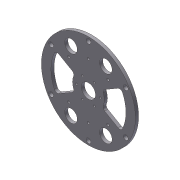
# Autodesk Inventor part: FlyWheel_Base_Jan21
Saved by Autodesk Inventor 2012 (Build 160160000, 160)
## iProperties
Created: 2012-01-22
Part Number: FlyWheel_Base_Jan21
Material: Aluminum-6061
Document SubType Name: Modeling
Designer: JesseK
Density: 2.71 g/cm^3
Mass: 341.466 g
Surface Area: 506.466 cm^2
Volume: 126.002 cm^3
Author: JesseK
Autodesk Inventor part; units mm, degrees
ref_plane "YZ Plane" through (0, 0, 0) normal (1, 0, 0) x (0, 1, 0)
ref_plane "XZ Plane" through (0, 0, 0) normal (0, 1, 0) x (-1, 0, 0)
ref_plane "XY Plane" through (0, 0, 0) normal (0, 0, 1) x (1, 0, 0)
sketch "Sketch1" plane through (0, 0, 0) normal (0, 0, 1) x (1, 0, 0)
  circle A0 centre (0, 0) radius 94.2975
  circle A1 centre (0, 0) radius 14.2875
  dimension "d0" = 188.595
  dimension "d1" = 28.575
  constraints: 2 centre point, 2 coincident
  measures "d0" diameter of A0
  measures "d1" diameter of A1
extrude "Extrusion1" add sketch "Sketch1" along normal blind 6.35
sketch "Sketch2" plane through (0, 0, 6.35) normal (0, 0, 1) x (1, 0, 0)
  circle A0 centre (0, 0) radius 94.2975 projected
  circle A1 centre (0, 0) radius 23.8125 construction
  line L0 (0, 0) -> (-11.9063, 20.6222) construction
  line L1 (0, 0) -> (0, 23.8125) construction
  circle A2 centre (-11.9063, 20.6222) radius 2.0193
  dimension "d4" = 47.625
  dimension "d5" = 30
  dimension "d6" = 4.0386
  constraints: 4 end point, 2 centre point, 2 coincident, 2 point on circle, 1 vertical
  measures "d4" diameter of A1
  measures "d5" angle of L1 L0
  measures "d6" diameter of A2
extrude "Extrusion2" cut sketch "Sketch2" against normal through all contours A2
pattern_circular "Circular Pattern1" count 6 over 360 about axis through (0, 0, -10) along (0, 0, 1) of "Extrusion2"
sketch "Sketch6" plane through (0, 0, 0) normal (0, 0, -1) x (-1, 0, 0)
  circle A0 centre (0, 0) radius 94.2975 projected
  circle A1 centre (0, 0) radius 55.5625 construction
  line L0 (0, 0) -> (0, -55.5625) construction
  circle A2 centre (0, -55.5625) radius 2.4384
  circle A3 centre (0, 0) radius 14.2875 projected
  line L1 (0, 0) -> (-39.2886, -39.2886) construction
  line L2 (0, 0) -> (39.2886, -39.2886) construction
  circle A4 centre (-39.2886, -39.2886) radius 2.4384
  circle A5 centre (39.2886, -39.2886) radius 2.4384
  dimension "d32" = 111.125
  dimension "d37" = 45
  dimension "d38" = 4.8768
  constraints: 6 end point, 4 centre point, 4 coincident, 3 point on circle, 2 equal radius, 1 perpendicular, 1 vertical
  measures "d32" diameter of A1
  measures "d37" angle of L0 L1
  measures "d38" diameter of A2
extrude "Extrusion5" cut sketch "Sketch6" against normal up to next contours A2 | A4 | A5
pattern_circular "Circular Pattern4" count 2 over 360 about axis through (0, 0, -10) along (0, 0, 1) of "Extrusion5"
sketch "Sketch7" plane through (0, 0, 0) normal (0, 0, -1) x (-1, 0, 0)
  circle A0 centre (0, 0) radius 94.2975 projected
  circle A1 centre (0, 0) radius 86.5188 construction
  circle A2 centre (0, -86.5188) radius 4.7625
  line L0 (0, -86.5188) -> (0, 0) construction
  dimension "d42" = 173.0375
  dimension "d43" = 9.525
  constraints: 2 end point, 1 centre point, 1 coincident, 1 vertical, 1 vertical alignment, 2 other
  measures "d43" diameter of A2
extrude "Extrusion6" cut sketch "Sketch7" against normal through all contours A2
pattern_circular "Circular Pattern5" count 6 over 360 about axis through (0, 0, -10) along (0, 0, 1) of "Extrusion6"
sketch "Sketch8" plane through (0, 0, 0) normal (0, 0, -1) x (-1, 0, 0)
  circle A0 centre (0, 0) radius 94.2975 projected
  arc A1 (-29.7576, 11.0702) -> (-29.7576, -11.0702) centre (0, 0) ccw
  arc A2 (-68.3565, 31.4575) -> (-68.3565, -31.4575) centre (0, 0) ccw
  line L0 (-59.413, 34.3021) -> (-32.5341, 18.7836)
  line L1 (-59.413, -34.3021) -> (-32.5341, -18.7836)
  line L2 (-27.4963, -15.875) -> (0, 0) construction
  line L3 (0, 0) -> (-27.4963, 15.875) construction
  line L4 (0, 0) -> (-75.2475, 0) construction
  line L5 (-65.1662, 37.6237) -> (-75.2475, 0) construction
  line L6 (-75.2475, 0) -> (-65.1662, -37.6237) construction
  arc A3 (-59.413, 34.3021) -> (-68.3565, 31.4575) centre (-62.588, 28.8029) ccw
  arc A4 (-29.7576, 11.0702) -> (-32.5341, 18.7836) centre (-35.7091, 13.2843) ccw
  arc A5 (-32.5341, -18.7836) -> (-29.7576, -11.0702) centre (-35.7091, -13.2843) ccw
  arc A6 (-68.3565, -31.4575) -> (-59.413, -34.3021) centre (-62.588, -28.8029) ccw
  dimension "d49" = 19.05
  dimension "d50" = 31.75
  dimension "d51" = 60
  dimension "d54" = 6.35
  constraints: 17 point on circle, 14 end point, 8 tangent, 6 centre point, 4 point on line, 3 equal radius, 2 coincident, 2 collinear, 1 equal length, 1 horizontal
  measures "d49" radial gap between concentric circles of A0 A2
  measures "d50" radius of A1
  measures "d51" angle of L1 L0
  measures "d54" radius of A3
extrude "Extrusion7" cut sketch "Sketch8" against normal through all contours A1 A5 L1 A6 A2 A3 L0 A4
pattern_circular "Circular Pattern6" count 2 over 360 about axis through (0, 0, -10) along (0, 0, 1) of "Extrusion7"
sketch "Sketch9" plane through (0, 0, 0) normal (0, 0, -1) x (-1, 0, 0)
  arc A0 (29.7576, -11.0702) -> (29.7576, 11.0702) centre (0, 0) ccw projected
  circle A1 centre (0, 0) radius 94.2975 projected
  circle A2 centre (0, 0) radius 69.85 construction
  line L0 (0, 0) -> (-34.925, 60.4919) construction
  line L1 (0, 0) -> (0, 69.85) construction
  circle A3 centre (-34.925, 60.4919) radius 12.7
  circle A4 centre (0, 0) radius 14.2875 projected
  line L2 (0, 0) -> (34.925, 60.4919) construction
  circle A5 centre (34.925, 60.4919) radius 12.7
  dimension "d59" = 25.4
  dimension "d60" = 30
  dimension "d66" = 30
  dimension "d67" = 139.7
  constraints: 6 end point, 4 coincident, 3 centre point, 3 point on circle, 1 equal radius, 1 vertical
  measures "d59" diameter of A3
  measures "d60" angle of L1 L0
  measures "d66" angle of L2 L1
  measures "d67" diameter of A2
extrude "Extrusion8" cut sketch "Sketch9" against normal through all contours A3 | A5
pattern_circular "Circular Pattern7" count 2 over 360 about axis through (0, 0, -10) along (0, 0, 1) of "Extrusion8"
body "Solid1"
